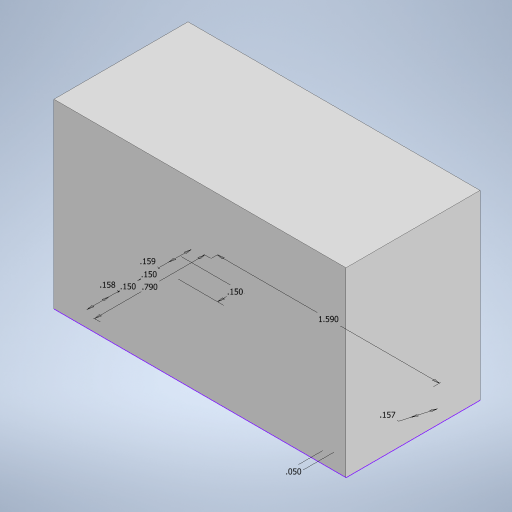
# Autodesk Inventor part: Servo Mount and Screw Hole Test
Saved by Autodesk Inventor 2023 (Build 270158000, 158)
## iProperties
Created: 2023-03-13
Part Number: Servo Mount and Screw Hole Test
Material: Generic
Document SubType Name: Modeling
Designer: tommy
Density: 1 g/cm^3
Appearance: Default
Author: tommy
Autodesk Inventor part; units mm, degrees
ref_plane "YZ Plane" through (0, 0, 0) normal (1, 0, 0) x (0, 1, 0)
ref_plane "XZ Plane" through (0, 0, 0) normal (0, 1, 0) x (-1, 0, 0)
ref_plane "XY Plane" through (0, 0, 0) normal (0, 0, 1) x (1, 0, 0)
sketch "Sketch1" plane through (0, 0, 0) normal (0, 1, 0) x (-1, 0, 0)
  line L0 (0, 0) -> (40.386, 0)
  line L1 (40.386, 0) -> (40.386, -20.066)
  line L2 (40.386, -20.066) -> (0, -20.066)
  line L3 (0, -20.066) -> (0, 0)
  line L4 (-6.35, 2.1529) -> (-6.35, -22.2189)
  line L5 (46.736, -22.2189) -> (46.736, 2.1529)
  line L6 (46.736, 2.1529) -> (-6.35, 2.1529)
  line L7 (-6.35, -22.2189) -> (46.736, -22.2189)
  circle A0 centre (43.6467, -2.7645) radius 2.0066
  circle A1 centre (43.6467, -17.653) radius 2.0193
  circle A2 centre (-3.3147, -15.0991) radius 1.9939
  line L8 (-1.27, -0.7579) -> (-3.8376, -0.7579)
  line L9 (-3.8376, -0.7579) -> (-3.8376, -4.7711)
  line L10 (-3.8376, -4.7711) -> (-1.27, -4.7711)
  line L11 (-1.27, -4.7711) -> (-1.27, -0.7579)
  line L12 (40.386, -10.033) -> (46.736, -10.033)
  line L13 (40.386, -13.843) -> (46.736, -13.843)
  line L14 (40.386, -6.223) -> (46.736, -6.223)
  dimension "d0" = 40.386
  dimension "d1" = 20.066
  dimension "d3" = 4.0132
  dimension "d4" = 4.0386
  dimension "d5" = 3.9878
  dimension "d6" = 3.81
  dimension "d7" = 3.81
  dimension "d8" = 3.81
  dimension "d9" = 1.27
  constraints: 30 end point, 8 parallel, 3 centre point, 2 horizontal, 2 midpoint, 2 perpendicular
  measures "d0" distance of L1.end L2.end
  measures "d1" distance of L0.end L1.end
  measures "d3" diameter of A0
  measures "d4" diameter of A1
  measures "d5" diameter of A2
  measures "d6" distance between parallel lines of L12 L13
  measures "d7" distance between parallel lines of L12 L14
  measures "d8" distance from line of L13 A1.centre
  measures "d9" distance between parallel lines of L3 L11
extrude "Extrusion1" add sketch "Sketch1" along normal blind 33.02 contours L3 L2 L1 L13 L5 L7 L4 L6 L14 L0 | L0 L1 L2 L3 | L14 L5 L12 L1 | L12 L5 L13 L1 | A0 | A1 | A2 | L11 L10 L9 L8
extrude "Extrusion2" cut sketch "Sketch1" along normal blind 24.638 contours L14 L5 L12 L1 | L12 L5 L13 L1 | A0 | A1 | A2 | L11 L10 L9 L8
extrude "Extrusion3" cut sketch "Sketch1" along normal blind 29.845 contours L0 L1 L2 L3
body "Solid1"
